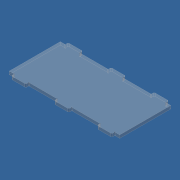
# Autodesk Inventor part: P1704_004
Saved by Autodesk Inventor 2015 (Build 190159000, 159)
## iProperties
Created: 2017-02-08
Part Number: P1704_004
Project: Polymanette chevalier
Material: Plastique PMMA
Description: Paroi latérale
Document SubType Name: Modeling
Designer: Alexandre.PICOTTE
Authority: 112.4x58x3
Density: 1.188 g/cm^3
Appearance: Transparent - Clair
Mass: 21.7466 g
Surface Area: 133.256 cm^2
Volume: 18.3052 cm^3
Material number: ---
Author: Boris.GAUDARD
Autodesk Inventor part; units mm, degrees
ref_plane "Plan YZ" through (0, 0, 0) normal (1, 0, 0) x (0, 1, 0)
ref_plane "Plan XZ" through (0, 0, 0) normal (0, 1, 0) x (-1, 0, 0)
ref_plane "Plan XY" through (0, 0, 0) normal (0, 0, 1) x (1, 0, 0)
sketch "Esquisse7" plane through (0, 0, 0) normal (0, 0, 1) x (1, 0, 0)
  line L0 (-56.2, -26) -> (-56.2, 26)
  line L1 (-56.2, 26) -> (-51.2, 26)
  line L2 (-51.2, 26) -> (-51.2, 29)
  line L3 (-51.2, 29) -> (-36.2, 29)
  line L4 (-36.2, 29) -> (-36.2, 26)
  line L5 (36.2, 26) -> (36.2, 29)
  line L6 (36.2, 29) -> (51.2, 29)
  line L7 (51.2, 29) -> (51.2, 26)
  line L8 (51.2, 26) -> (56.2, 26)
  line L9 (56.2, 26) -> (56.2, -26)
  line L10 (56.2, -26) -> (51.2, -26)
  line L11 (51.2, -26) -> (51.2, -29)
  line L12 (51.2, -29) -> (36.2, -29)
  line L13 (36.2, -29) -> (36.2, -26)
  line L14 (-36.2, -26) -> (-36.2, -29)
  line L15 (-51.2, -29) -> (-51.2, -26)
  line L16 (-56.2, -26) -> (-51.2, -26)
  line L17 (-51.2, -29) -> (-36.2, -29)
  line L18 (0, -40.6) -> (0, 40.6) construction
  line L19 (-78.68, 0) -> (78.68, 0) construction
  line L20 (7.5, 26) -> (7.5, 29)
  line L21 (7.5, 29) -> (-7.5, 29)
  line L22 (-7.5, 29) -> (-7.5, 26)
  line L23 (7.5, -26) -> (7.5, -29)
  line L24 (7.5, -29) -> (-7.5, -29)
  line L25 (-7.5, -29) -> (-7.5, -26)
  line L26 (-36.2, -26) -> (-7.5, -26)
  line L27 (7.5, -26) -> (36.2, -26)
  line L28 (-36.2, 26) -> (-7.5, 26)
  line L29 (7.5, 26) -> (36.2, 26)
  point P0 (0, 0)
  dimension "d33" = 52
  dimension "d34" = 5
  dimension "d35" = 3
  dimension "d36" = 15
  dimension "d51" = 112.4
  constraints: 56 end point, 17 point on line, 10 perpendicular, 6 equal length, 5 parallel, 4 collinear, 2 horizontal, 1 vertical, 3 other
  measures "d33" distance of L0.start L0.end
  measures "d34" distance of L0.end L1.end
  measures "d35" distance of L1.end L2.end
  measures "d36" distance of L2.end L3.end
  measures "d51" distance between parallel lines of L9 L0
extrude "Extrusion2" add sketch "Esquisse7" along normal blind 3
chamfer "Chanfrein4" distance 1 angle 45 12 edges at (-51.2, 29, 1.5) (-7.5, 29, 1.5) (36.2, 29, 1.5) (-36.2, 29, 1.5) (7.5, 29, 1.5) (51.2, 29, 1.5) (-36.2, -29, 1.5) (-51.2, -29, 1.5) (-7.5, -29, 1.5) (7.5, -29, 1.5) (36.2, -29, 1.5) (51.2, -29, 1.5)
sketch "Esquisse9" plane through (0, 0, 3) normal (0, 0, 1) x (1, 0, 0)
  line L0 (-56.2, 26) -> (-51.2, 26) construction
  line L1 (-51.2, 26) -> (-51.2, 28) construction
  line L2 (-36.2, 28) -> (-36.2, 26) construction
  line L3 (-36.2, 26) -> (-7.5, 26) construction
  line L4 (-7.5, 26) -> (-7.5, 28) construction
  line L5 (7.5, 28) -> (7.5, 26) construction
  line L6 (7.5, 26) -> (36.2, 26) construction
  line L7 (36.2, 26) -> (36.2, 28) construction
  line L8 (51.2, 28) -> (51.2, 26) construction
  line L9 (51.2, 26) -> (56.2, 26) construction
  line L10 (7.5, -26) -> (7.5, -28) construction
  line L11 (36.2, -26) -> (7.5, -26) construction
  line L12 (36.2, -28) -> (36.2, -26) construction
  line L13 (51.2, -26) -> (51.2, -28) construction
  line L14 (56.2, -26) -> (51.2, -26) construction
  line L15 (-7.5, -26) -> (-36.2, -26) construction
  line L16 (-7.5, -28) -> (-7.5, -26) construction
  line L17 (-36.2, -26) -> (-36.2, -28) construction
  line L18 (-51.2, -28) -> (-51.2, -26) construction
  line L19 (-51.2, -26) -> (-56.2, -26) construction
  point P0 (0, 0)
  constraints: 12 coincident
hole "Perçage3" at (-51.2, 26, 3) at (-36.2, 26, 3) at (-7.5, 26, 3) at (36.2, 26, 3) at (51.2, 26, 3) at (7.5, 26, 3) at (36.2, -26, 3) at (51.2, -26, 3) at (7.5, -26, 3) at (-7.5, -26, 3) at (-36.2, -26, 3) at (-51.2, -26, 3) direction (0, 0, -1) diameter 1 end through all
